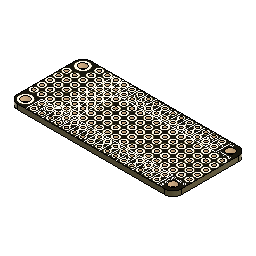
2884 Proto FeatherWing (Autodesk Fusion 360 design; units mm, degrees)
part number: FEATHERWING
Autodesk Fusion 360 part; units mm, degrees
sketch "sketch 280" plane through (0, 0, 0) normal (0, 0, 1) x (1, 0, 0)
  line L0 (2.54, 22.86) -> (48.26, 22.86)
  arc A0 (50.8, 20.32) -> (48.26, 22.86) centre (48.26, 20.32) ccw
  line L1 (50.8, 20.32) -> (50.8, 2.54)
  arc A1 (48.26, 0) -> (50.8, 2.54) centre (48.26, 2.54) ccw
  line L2 (48.26, 0) -> (2.54, 0)
  arc A2 (0, 2.54) -> (2.54, 0) centre (2.54, 2.54) ccw
  line L3 (0, 2.54) -> (0, 20.32)
  arc A3 (2.54, 22.86) -> (0, 20.32) centre (2.54, 20.32) ccw
  line L4 (2.54, 0) -> (48.26, 0)
  arc A4 (48.26, 0) -> (50.8, 2.54) centre (48.26, 2.54) ccw
  line L5 (50.8, 2.54) -> (50.8, 20.32)
  arc A5 (50.8, 20.32) -> (48.26, 22.86) centre (48.26, 20.32) ccw
  line L6 (48.26, 22.86) -> (2.54, 22.86)
  arc A6 (2.54, 22.86) -> (0, 20.32) centre (2.54, 20.32) ccw
  line L7 (0, 20.32) -> (0, 2.54)
  arc A7 (0, 2.54) -> (2.54, 0) centre (2.54, 2.54) ccw
extrude "Board" add sketch "sketch 280" along normal blind 1.57 makes body 1 in component "Board"
sketch "sketch 1543" plane through (0, 0, 0) normal (0, 0, 1) x (1, 0, 0)
  line L0 (1.29, 0.77) -> (49.53, 0.77)
  line L1 (49.53, 0.77) -> (49.53, 22.09)
  line L2 (49.53, 22.09) -> (1.29, 22.09)
  line L3 (1.29, 22.09) -> (1.29, 0.77)
extrude "FEATHERWING" add sketch "sketch 1543" along normal blind 0.1 separate body makes body 2 in component "FEATHERWING"
sketch "sketch 1674" plane through (0, 0, 0) normal (0, 0, 1) x (1, 0, 0)
  line L0 (-19.55, -0.5) -> (19.55, -0.5)
  line L1 (19.55, -0.5) -> (19.55, 0.5)
  line L2 (19.55, 0.5) -> (-19.55, 0.5)
  line L3 (-19.55, 0.5) -> (-19.55, -0.5)
extrude "1X16_ROUND_76MIL" add sketch "sketch 1674" along normal blind 0.1 separate body makes body 3 in component "1X16_ROUND_76MIL"
sketch "sketch 1805" plane through (0, 0, 0) normal (0, 0, 1) x (1, 0, 0)
  line L0 (-15.24, -0.635) -> (14.47, -0.635)
  line L1 (14.47, -0.635) -> (14.47, 0.635)
  line L2 (14.47, 0.635) -> (-15.24, 0.635)
  line L3 (-15.24, 0.635) -> (-15.24, -0.635)
extrude "1X12_ROUND_76MIL" add sketch "sketch 1805" along normal blind 0.1 separate body makes body 4 in component "1X12_ROUND_76MIL"
sketch "sketch 424" plane through (0, 0, 0) normal (0, 0, 1) x (1, 0, 0)
  circle A0 centre (13.97, 6.35) radius 0.6
  circle A1 centre (13.97, 8.89) radius 0.6
  circle A2 centre (13.97, 11.43) radius 0.6
  circle A3 centre (13.97, 13.97) radius 0.6
  circle A4 centre (13.97, 16.51) radius 0.6
  circle A5 centre (13.97, 19.05) radius 0.6
  circle A6 centre (13.97, 21.59) radius 0.6
  circle A7 centre (11.43, 6.35) radius 0.6
  circle A8 centre (11.43, 8.89) radius 0.6
  circle A9 centre (11.43, 11.43) radius 0.6
  circle A10 centre (11.43, 13.97) radius 0.6
  circle A11 centre (11.43, 16.51) radius 0.6
  circle A12 centre (11.43, 19.05) radius 0.6
  circle A13 centre (11.43, 21.59) radius 0.6
  circle A14 centre (8.89, 21.59) radius 0.6
  circle A15 centre (8.89, 19.05) radius 0.6
  circle A16 centre (6.35, 19.05) radius 0.6
  circle A17 centre (6.35, 21.59) radius 0.6
  circle A18 centre (6.35, 16.51) radius 0.6
  circle A19 centre (3.81, 16.51) radius 0.6
  circle A20 centre (1.27, 16.51) radius 0.6
  circle A21 centre (1.27, 13.97) radius 0.6
  circle A22 centre (3.81, 13.97) radius 0.6
  circle A23 centre (6.35, 13.97) radius 0.6
  circle A24 centre (6.35, 11.43) radius 0.6
  circle A25 centre (3.81, 11.43) radius 0.6
  circle A26 centre (1.27, 11.43) radius 0.6
  circle A27 centre (1.27, 8.89) radius 0.6
  circle A28 centre (3.81, 8.89) radius 0.6
  circle A29 centre (6.35, 8.89) radius 0.6
  circle A30 centre (6.35, 6.35) radius 0.6
  circle A31 centre (3.81, 6.35) radius 0.6
  circle A32 centre (1.27, 6.35) radius 0.6
  circle A33 centre (8.89, 6.35) radius 0.6
  circle A34 centre (8.89, 8.89) radius 0.6
  circle A35 centre (8.89, 11.43) radius 0.6
  circle A36 centre (8.89, 13.97) radius 0.6
  circle A37 centre (8.89, 16.51) radius 0.6
  circle A38 centre (16.51, 16.51) radius 0.6
  circle A39 centre (19.05, 16.51) radius 0.6
  circle A40 centre (21.59, 16.51) radius 0.6
  circle A41 centre (16.51, 13.97) radius 0.6
  circle A42 centre (16.51, 11.43) radius 0.6
  circle A43 centre (16.51, 8.89) radius 0.6
  circle A44 centre (16.51, 6.35) radius 0.6
  circle A45 centre (19.05, 6.35) radius 0.6
  circle A46 centre (19.05, 8.89) radius 0.6
  circle A47 centre (19.05, 11.43) radius 0.6
  circle A48 centre (19.05, 13.97) radius 0.6
  circle A49 centre (21.59, 13.97) radius 0.6
  circle A50 centre (21.59, 11.43) radius 0.6
  circle A51 centre (21.59, 8.89) radius 0.6
  circle A52 centre (21.59, 6.35) radius 0.6
  circle A53 centre (24.13, 6.35) radius 0.6
  circle A54 centre (24.13, 8.89) radius 0.6
  circle A55 centre (24.13, 16.51) radius 0.6
  circle A56 centre (24.13, 13.97) radius 0.6
  circle A57 centre (24.13, 11.43) radius 0.6
  circle A58 centre (26.67, 6.35) radius 0.6
  circle A59 centre (26.67, 8.89) radius 0.6
  circle A60 centre (26.67, 11.43) radius 0.6
  circle A61 centre (26.67, 13.97) radius 0.6
  circle A62 centre (26.67, 16.51) radius 0.6
  circle A63 centre (29.21, 16.51) radius 0.6
  circle A64 centre (29.21, 13.97) radius 0.6
  circle A65 centre (29.21, 11.43) radius 0.6
  circle A66 centre (29.21, 8.89) radius 0.6
  circle A67 centre (29.21, 6.35) radius 0.6
  circle A68 centre (31.75, 6.35) radius 0.6
  circle A69 centre (31.75, 8.89) radius 0.6
  circle A70 centre (31.75, 11.43) radius 0.6
  circle A71 centre (31.75, 13.97) radius 0.6
  circle A72 centre (31.75, 16.51) radius 0.6
  circle A73 centre (34.29, 16.51) radius 0.6
  circle A74 centre (34.29, 13.97) radius 0.6
  circle A75 centre (34.29, 11.43) radius 0.6
  circle A76 centre (34.29, 8.89) radius 0.6
  circle A77 centre (34.29, 6.35) radius 0.6
  circle A78 centre (36.83, 6.35) radius 0.6
  circle A79 centre (36.83, 8.89) radius 0.6
  circle A80 centre (36.83, 11.43) radius 0.6
  circle A81 centre (36.83, 13.97) radius 0.6
  circle A82 centre (36.83, 16.51) radius 0.6
  circle A83 centre (39.37, 16.51) radius 0.6
  circle A84 centre (39.37, 13.97) radius 0.6
  circle A85 centre (39.37, 11.43) radius 0.6
  circle A86 centre (39.37, 8.89) radius 0.6
  circle A87 centre (39.37, 6.35) radius 0.6
  circle A88 centre (41.91, 6.35) radius 0.6
  circle A89 centre (41.91, 16.51) radius 0.6
  circle A90 centre (41.91, 13.97) radius 0.6
  circle A91 centre (41.91, 11.43) radius 0.6
  circle A92 centre (41.91, 8.89) radius 0.6
  circle A93 centre (44.45, 6.35) radius 0.6
  circle A94 centre (44.45, 8.89) radius 0.6
  circle A95 centre (44.45, 11.43) radius 0.6
  circle A96 centre (44.45, 13.97) radius 0.6
  circle A97 centre (44.45, 16.51) radius 0.6
  circle A98 centre (46.99, 16.51) radius 0.6
  circle A99 centre (49.53, 16.51) radius 0.6
  circle A100 centre (49.53, 13.97) radius 0.6
  circle A101 centre (49.53, 11.43) radius 0.6
  circle A102 centre (49.53, 8.89) radius 0.6
  circle A103 centre (49.53, 6.35) radius 0.6
  circle A104 centre (46.99, 6.35) radius 0.6
  circle A105 centre (46.99, 8.89) radius 0.6
  circle A106 centre (46.99, 11.43) radius 0.6
  circle A107 centre (46.99, 13.97) radius 0.6
  circle A108 centre (48.26, 20.32) radius 1.27
  circle A109 centre (48.26, 2.54) radius 1.27
  circle A110 centre (2.54, 20.32) radius 1.25
  circle A111 centre (2.54, 2.54) radius 1.25
  circle A112 centre (16.51, 21.59) radius 0.5
  circle A113 centre (19.05, 21.59) radius 0.5
  circle A114 centre (21.59, 21.59) radius 0.5
  circle A115 centre (24.13, 21.59) radius 0.5
  circle A116 centre (26.67, 21.59) radius 0.5
  circle A117 centre (29.21, 21.59) radius 0.5
  circle A118 centre (31.75, 21.59) radius 0.5
  circle A119 centre (34.29, 21.59) radius 0.5
  circle A120 centre (36.83, 21.59) radius 0.5
  circle A121 centre (39.37, 21.59) radius 0.5
  circle A122 centre (41.91, 21.59) radius 0.5
  circle A123 centre (44.45, 21.59) radius 0.5
  circle A124 centre (16.51, 1.27) radius 0.5
  circle A125 centre (19.05, 1.27) radius 0.5
  circle A126 centre (21.59, 1.27) radius 0.5
  circle A127 centre (24.13, 1.27) radius 0.5
  circle A128 centre (26.67, 1.27) radius 0.5
  circle A129 centre (29.21, 1.27) radius 0.5
  circle A130 centre (31.75, 1.27) radius 0.5
  circle A131 centre (34.29, 1.27) radius 0.5
  circle A132 centre (36.83, 1.27) radius 0.5
  circle A133 centre (39.37, 1.27) radius 0.5
  circle A134 centre (41.91, 1.27) radius 0.5
  circle A135 centre (44.45, 1.27) radius 0.5
  circle A136 centre (13.97, 1.27) radius 0.5
  circle A137 centre (11.43, 1.27) radius 0.5
  circle A138 centre (8.89, 1.27) radius 0.5
  circle A139 centre (6.35, 1.27) radius 0.5
  circle A140 centre (44.45, 3.81) radius 0.5
  circle A141 centre (41.91, 3.81) radius 0.5
  circle A142 centre (39.37, 3.81) radius 0.5
  circle A143 centre (36.83, 3.81) radius 0.5
  circle A144 centre (34.29, 3.81) radius 0.5
  circle A145 centre (31.75, 3.81) radius 0.5
  circle A146 centre (29.21, 3.81) radius 0.5
  circle A147 centre (26.67, 3.81) radius 0.5
  circle A148 centre (24.13, 3.81) radius 0.5
  circle A149 centre (21.59, 3.81) radius 0.5
  circle A150 centre (19.05, 3.81) radius 0.5
  circle A151 centre (16.51, 3.81) radius 0.5
  circle A152 centre (13.97, 3.81) radius 0.5
  circle A153 centre (11.43, 3.81) radius 0.5
  circle A154 centre (8.89, 3.81) radius 0.5
  circle A155 centre (6.35, 3.81) radius 0.5
  circle A156 centre (16.51, 19.05) radius 0.5
  circle A157 centre (19.05, 19.05) radius 0.5
  circle A158 centre (21.59, 19.05) radius 0.5
  circle A159 centre (24.13, 19.05) radius 0.5
  circle A160 centre (26.67, 19.05) radius 0.5
  circle A161 centre (29.21, 19.05) radius 0.5
  circle A162 centre (31.75, 19.05) radius 0.5
  circle A163 centre (34.29, 19.05) radius 0.5
  circle A164 centre (36.83, 19.05) radius 0.5
  circle A165 centre (39.37, 19.05) radius 0.5
  circle A166 centre (41.91, 19.05) radius 0.5
  circle A167 centre (44.45, 19.05) radius 0.5
extrude "Extrude2" cut sketch "sketch 424" along normal blind 1.57 bodies 1 in component "Board"
component "Board" placed x (1, 0, 0) y (0, 1, 0) z (0, 0, 1) at (0, 0, 0)
component "FEATHERWING" placed x (1, 0, 0) y (0, 1, 0) z (0, 0, 1) at (0, 0, 1.57)
component "1X16_ROUND_76MIL" placed x (-1, 0, 0) y (0, -1, 0) z (0, 0, 1) at (25.4, 3.81, 1.57)
component "1X12_ROUND_76MIL" placed x (1, 0, 0) y (0, 1, 0) z (0, 0, 1) at (30.48, 19.05, 1.57)
named bodies: "Board", "FEATHERWING", "1X16_ROUND_76MIL", "1X12_ROUND_76MIL"
